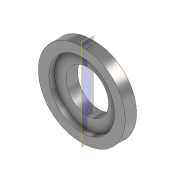
# Autodesk Inventor part: Tilting head - cover side part
Saved by Autodesk Inventor 2020.3 (Build 243373010, 373A)
## iProperties
Created: 2021-05-11
Part Number: Tilting head - cover side part
Material: Steel, Carbon
Document SubType Name: Modeling
Designer: marti
Density: 7.85 g/cm^3
Appearance: Semi-Polished
Author: marti
Autodesk Inventor part; units mm, degrees
ref_plane "YZ Plane" through (0, 0, 0) normal (1, 0, 0) x (0, 1, 0)
ref_plane "XZ Plane" through (0, 0, 0) normal (0, 1, 0) x (-1, 0, 0)
ref_plane "XY Plane" through (0, 0, 0) normal (0, 0, 1) x (1, 0, 0)
sketch "Sketch1" plane through (0, 0, 0) normal (0, 0, 1) x (1, 0, 0)
  circle A0 centre (0, 0) radius 28.75
  line L0 (3.5274, -36.2072) -> (-3.5274, -36.2072)
  line L1 (-3.5274, 36.2072) -> (3.5274, 36.2072)
  arc A1 (3.5274, -36.2072) -> (3.5274, 36.2072) centre (1.7656, 0) ccw
  arc A2 (-3.5274, 36.2072) -> (-3.5274, -36.2072) centre (-1.7656, 0) ccw
  line L2 (3.3345, -28.7072) -> (-3.3345, -28.7072)
  point P0 (0, 0)
  point P1 (0, 36.2072)
  point P2 (0, 0)
  point P3 (0, -28.7072)
  dimension "d0" = 57.5
  dimension "d1" = 36.25
  dimension "d2" = 36.25
  dimension "d8" = 7.0549
  constraints: 6 end point, 4 point on circle, 3 centre point, 2 midpoint, 2 vertical alignment, 1 coincident, 1 horizontal alignment
  measures "d0" diameter of A0
  measures "d1" radius of A1
  measures "d2" radius of A2
  measures "d8" distance of L1.start L1.end
extrude "Extrusion1" add sketch "Sketch1" along normal mid plane 10
sketch "Sketch2" plane through (0, 0, 0) normal (0, 0, 1) x (1, 0, 0)
  circle A0 centre (0, 0) radius 28.75 projected
  circle A1 centre (0, 0) radius 18.5625
  dimension "d5" = 37.125
  constraints: 1 centre point, 1 coincident
  measures "d5" diameter of A1
extrude "Extrusion2" add sketch "Sketch2" against normal blind 10
ref_plane "Work Plane1" through (0, 36.2072, 5) normal (-1, 0, 0) x (0, 0, -1)
body "Solid1"
